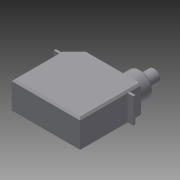
# Autodesk Inventor part: HD1440A_Servo
Saved by Autodesk Inventor 2015 (Build 190159000, 159)
## iProperties
Created: 2015-02-11
Part Number: HD1440A_Servo
Material: Generic
Document SubType Name: Modeling
Designer: Judson
Density: 1 g/cm^3
Appearance: Default
Author: Judson
Autodesk Inventor part; units mm, degrees
ref_plane "YZ Plane" through (0, 0, 0) normal (1, 0, 0) x (0, 1, 0)
ref_plane "XZ Plane" through (0, 0, 0) normal (0, 1, 0) x (-1, 0, 0)
ref_plane "XY Plane" through (0, 0, 0) normal (0, 0, 1) x (1, 0, 0)
sketch "Sketch1" plane through (0, 0, 0) normal (0, 1, 0) x (-1, 0, 0)
  line L0 (7.8024, -7.4673) -> (-12.3976, -7.4673)
  line L1 (-12.3976, -7.4673) -> (-12.3976, 14.7327)
  line L2 (-12.3976, 14.7327) -> (7.8024, 14.7327)
  line L3 (7.8024, 14.7327) -> (7.8024, -7.4673)
  line L4 (-12.3976, 0.0327) -> (7.8024, 0.0327)
  line L5 (-12.3976, -3.7208) -> (4.0489, -3.7208)
  line L6 (7.8024, 0.0327) -> (4.0489, -3.7208)
  point P0 (0, 0)
  dimension "d0" = 20.2
  dimension "d1" = 22.2
  dimension "d2" = 14.7
  dimension "d3" = 7.5
  dimension "d4" = 3.7465
  dimension "d5" = 45
  constraints: 14 end point, 3 point on line, 2 horizontal, 2 parallel, 2 perpendicular
  measures "d0" distance of L0.start L0.end
  measures "d1" distance of L2.end L0.start
  measures "d2" distance between parallel lines of L2 L4
  measures "d3" distance of L4.start L0.end
  measures "d4" distance between parallel lines of L0 L5
  measures "d5" angle of L4 L6
extrude "Extrusion1" add sketch "Sketch1" along normal blind 8.5 contours L4 L1 L2 L3 | L6 L5 L1 L4
chamfer "Chamfer1" distance 0.508 angle 45 1 edges at (12.3976, 8.5, 5.506)
chamfer "Chamfer2" distance 0.508 angle 45 1 edges at (3.9204, 8.5, -3.7208)
chamfer "Chamfer3" distance 0.508 angle 45 1 edges at (-7.8024, 8.5, 7.3827)
chamfer "Chamfer4" distance 0.508 angle 45 1 edges at (-5.9256, 8.5, -1.844)
chamfer "Chamfer5" distance 0.508 angle 45 1 edges at (2.2976, 8.5, 14.7327)
chamfer "Chamfer6" distance 0.508 angle 45 5 edges at (-5.9256, 0, -1.844) (-7.8024, 0, 7.3827) (2.2976, 0, 14.7327) (12.3976, 0, 5.506) (4.1744, 0, -3.7208)
sketch "Sketch2" plane through (-7.8024, 7.992, 0.0327) normal (-1, 0, 0) x (0, 0, 1)
  line L0 (0, 0) -> (14.7, 0) projected
  line L1 (0, -7.484) -> (0.635, -7.484)
  line L2 (0.635, -7.484) -> (0.635, 0)
  line L3 (0.635, 0) -> (0, 0)
  line L4 (0, 0) -> (0, -7.484)
  point P0 (-0.0327, -7.992)
  point P1 (14.7, 0)
  point P2 (1.5266, 1.0795)
  point P3 (13.6205, 0)
  dimension "d26" = 0.635
  constraints: 8 end point, 2 parallel, 1 horizontal, 1 perpendicular, 2 other
  measures "d26" distance of point (0, 0) L2.end
extrude "Extrusion2" add sketch "Sketch2" along normal blind 1.65 and the other way blind 21.85
chamfer "Chamfer7" distance 0.508 angle 45 1 edges at (12.3976, 4.25, -3.7208)
sketch "Sketch4" plane through (-4.0489, 0.508, -3.7208) normal (0, 0, -1) x (-1, 0, 0)
  line L0 (-15.9385, 0) -> (-15.9385, 7.484) projected
  line L1 (0, 0) -> (-15.9385, 0) projected
  line L2 (0, 0) -> (0, 7.484) projected
  line L3 (-15.9385, 7.484) -> (0, 7.484) projected
  line L4 (0, 0) -> (-15.9385, 0) projected
  circle A0 centre (-12.1965, 3.742) radius 3.742
  point P0 (-4.0489, -0.508)
  constraints: 3 tangent, 1 centre point
extrude "Extrusion3" add sketch "Sketch4" along normal blind 3.75 contours A0
chamfer "Chamfer8" distance 0.508 angle 45 1 edges at (11.8896, 4.25, -7.4708)
sketch "Sketch5" plane through (8.1476, 4.25, -7.4708) normal (0, 0, -1) x (-1, 0, 0)
  circle A0 centre (0, 0) radius 3.234 projected
  circle A1 centre (0, 0) radius 1.905
  point P0 (8.1476, -4.25)
  dimension "d39" = 3.81
  constraints: 1 centre point, 1 coincident
  measures "d39" diameter of A1
extrude "Extrusion4" add sketch "Sketch5" along normal blind 3.8382 contours A1
sketch "Sketch6" plane through (-4.0489, 0.508, -3.7208) normal (0, 0, -1) x (-1, 0, 0)
  circle A0 centre (-12.1965, 3.742) radius 1.905 projected
  point P0 (-4.0489, -0.508)
sketch "Sketch7" plane through (-4.0489, 0.508, -3.7208) normal (0, 0, -1) x (-1, 0, 0)
  arc A0 (-12.1965, 0) -> (-12.1965, 7.484) centre (-12.1965, 3.742) ccw projected
  line L0 (0, 0) -> (-12.1965, 0) projected
  line L1 (0, 0) -> (0, 7.484) projected
  line L2 (-12.1965, 7.484) -> (0, 7.484) projected
  circle A1 centre (-12.1965, 3.742) radius 1.905 projected
  circle A2 centre (-12.1965, 3.742) radius 1.905 projected
  circle A3 centre (-12.1965, 3.742) radius 3.234 projected
  circle A4 centre (-12.1965, 3.742) radius 3.234 projected
  arc A5 (-12.1965, 7.484) -> (-15.9385, 3.742) centre (-12.1965, 3.742) ccw projected
  line L3 (-15.9385, 7.484) -> (-12.1965, 7.484) projected
  line L4 (-15.9385, 3.742) -> (-15.9385, 7.484) projected
  line L5 (-15.9385, 3.742) -> (-15.9385, 7.484) projected
  line L6 (-16.4465, 7.484) -> (-16.4465, 0) projected
  arc A6 (-15.9385, 3.742) -> (-12.1965, 0) centre (-12.1965, 3.742) ccw projected
  line L7 (-15.9385, 0) -> (-15.9385, 3.742) projected
  line L8 (-12.1965, 0) -> (-15.9385, 0) projected
  line L9 (-16.4465, 7.484) -> (-16.4465, 0) projected
  line L10 (-18.0965, 7.484) -> (-16.4465, 7.484) projected
  line L11 (-18.0965, 0) -> (-18.0965, 7.484) projected
  line L12 (-16.4465, 0) -> (-18.0965, 0) projected
  point P0 (-4.0489, -0.508)
  dimension "d42" = 5.9
  measures "d42" distance from line of A1.centre L11
body "Solid1"
